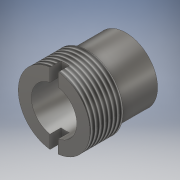
# Autodesk Inventor part: VS-005(COLLAR)
Saved by Autodesk Inventor 2017 SP1 (Build 210196100, 196)
## iProperties
Created: 2016-12-05
Part Number: VS-005(COLLAR)
Material: Steel, Carbon
Document SubType Name: Modeling
Designer: OCCC
Density: 7.85 g/cm^3
Appearance: Semi-Polished
Author: OCCC
Autodesk Inventor part; units mm, degrees
ref_plane "YZ Plane" through (0, 0, 0) normal (1, 0, 0) x (0, 1, 0)
ref_plane "XZ Plane" through (0, 0, 0) normal (0, 1, 0) x (-1, 0, 0)
ref_plane "XY Plane" through (0, 0, 0) normal (0, 0, 1) x (1, 0, 0)
sketch "Sketch1" plane through (0, 0, 0) normal (0, 0, 1) x (1, 0, 0)
  circle A0 centre (0, 0) radius 9.1281
  dimension "d0" = 18.2563
  dimension "d1" = 0
  constraints: 1 centre point
  measures "d0" diameter of A0
  measures "d1" distance of A0.centre point (0, 0)
extrude "Extrusion1" add sketch "Sketch1" against normal blind 11.1125
sketch "Sketch2" plane through (0, 0, 0) normal (0, 0, 1) x (1, 0, 0)
  circle A0 centre (0, 0) radius 10.3188
  dimension "d15" = 20.6375
  constraints: 1 centre point, 1 coincident
  measures "d15" diameter of A0
extrude "Extrusion2" add sketch "Sketch2" along normal blind 9.525
hole "Hole1" at (0, 0, 9.525) direction (0, 0, -1) diameter 13.0969 end through all
thread "Thread2" size "13/16-20 UNEF" class "2A" standard "ANSI Unified Screw Threads" length 9.525
sketch "Sketch3" plane through (0, 0, 9.525) normal (0, 0, 1) x (1, 0, 0)
  line L0 (0, -7.6975) -> (0, 10.1618) construction
  line L1 (0, 11.43) -> (1.1906, 11.43)
  line L2 (1.1906, 11.43) -> (1.1906, -11.43)
  line L3 (1.1906, -11.43) -> (0, -11.43)
  line L4 (0, 11.43) -> (-1.1906, 11.43)
  line L5 (-1.1906, 11.43) -> (-1.1906, -11.43)
  line L6 (-1.1906, -11.43) -> (0, -11.43)
  point P0 (0, 0)
  dimension "d22" = 1.1906
  dimension "d23" = 11.43
  dimension "d24" = 11.43
  constraints: 14 end point, 3 perpendicular, 3 point on line, 2 symmetric about line, 1 vertical
  measures "d22" distance of L1.start L1.end
  measures "d23" distance from line of point (0, 0) L1
  measures "d24" distance from line of L3 point (0, 0)
extrude "Extrusion3" cut sketch "Sketch3" against normal blind 3.175
body "Solid1"
